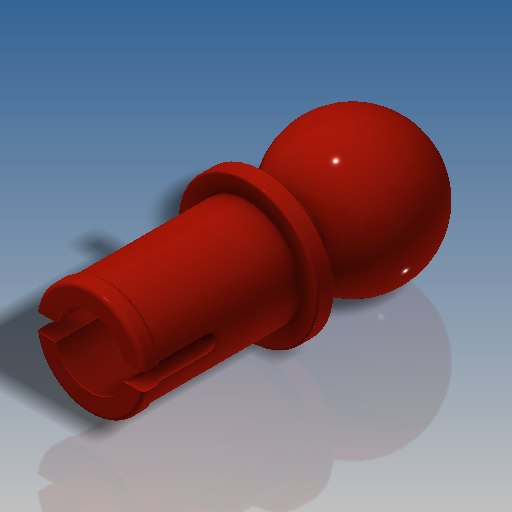
# Autodesk Inventor part: 6628-Red
Saved by Autodesk Inventor 2019.4 (Build 234330000, 330)
## iProperties
Created: 2014-06-03
Part Number: 6628-Red
Material: ABS Plastic
Document SubType Name: Modeling
Designer: D. Kohfeld
Appearance: Red
Density: 1.06 g/cm^3
Mass: 0.254458 g
Surface Area: 3.85266 cm^2
Volume: 0.240054 cm^3
Author: D. Kohfeld
Autodesk Inventor part; units mm, degrees
ref_plane "YZ Plane" through (0, 0, 0) normal (1, 0, 0) x (0, 1, 0)
ref_plane "XZ Plane" through (0, 0, 0) normal (0, 1, 0) x (-1, 0, 0)
ref_plane "XY Plane" through (0, 0, 0) normal (0, 0, 1) x (1, 0, 0)
sketch "Sketch1" plane through (0, 0, 0) normal (0, 1, 0) x (-1, 0, 0)
  line L0 (2.4, 7.2) -> (2.4, 0.8)
  line L1 (3.2, 0.8) -> (2.4, 0.8)
  line L2 (3.2, 0.8) -> (3.2, 0)
  line L3 (2.5, 8) -> (2.5, 7.2)
  line L4 (2.5, 8) -> (1.6, 8)
  line L5 (0, -10.9766) -> (0, 11.1628) projected
  line L6 (2.4, 7.2) -> (2.5, 7.2)
  line L7 (1.6, 8) -> (1.6, 0.8)
  line L8 (4.6692, 0) -> (-0.7782, 0) projected
  line L9 (1.6, 0.8) -> (0, 0.8)
  line L10 (0, -7.2) -> (0, 0.8)
  line L11 (3.2, 0) -> (1.6, 0)
  line L12 (1.6, 0) -> (1.6, -1.2287)
  arc A0 (0, -7.2) -> (1.6, -1.2287) centre (0, -4) ccw
  point P0 (0, 0)
  dimension "d1" = 4.8
  dimension "d2" = 5
  dimension "d6" = 8
  dimension "d7" = 0.8
  dimension "d8" = 6.4
  dimension "d9" = 0.8
  dimension "d32" = 6.4
  dimension "d33" = 4
  dimension "d34" = 3.2
  dimension "d37" = 3.2
  constraints: 22 end point, 5 point on line, 4 perpendicular, 2 point on circle, 1 centre point, 1 horizontal alignment, 1 parallel
  measures "d1" diameter of L0 L5
  measures "d2" diameter of L3 L5
  measures "d6" distance between parallel lines of L4 L8
  measures "d7" distance from line of L3.end L4
  measures "d8" diameter of L2 L5
  measures "d9" distance between parallel lines of L1 L8
  measures "d32" diameter of A0
  measures "d33" distance from line of L8 A0.centre
  measures "d34" diameter of L12 L5
  measures "d37" diameter of L7 L5
revolve "Revolution1" add sketch "Sketch1" angle 360 about axis through (0, 0, -10) along (0, 0, 1)
fillet "Fillet1" radius 0.2 2 edges at (2.5, 0, 8) (2.5, 0, 7.2)
fillet "Fillet1" radius 0.1 2 edges at (3.2, 0, 0) (3.2, 0, 0.8)
sketch "Sketch2" plane through (0, 0, 0) normal (1, 0, 0) x (0, 1, 0)
  line L0 (-1.6, 8) -> (1.6, 8) projected
  line L1 (-0.4, 8) -> (0.4, 8)
  line L2 (0.4, 8) -> (0.4, 5)
  line L3 (-0.4, 5) -> (-0.4, 8)
  arc A0 (-0.4, 5) -> (0.4, 5) centre (0, 5) ccw
  point P0 (0, 0)
  point P1 (0, 8)
  dimension "d35" = 3.4
  dimension "d36" = 0.8
  constraints: 6 end point, 2 midpoint, 2 point on circle, 2 tangent, 1 centre point, 1 horizontal, 1 parallel, 1 perpendicular, 1 point on line
  measures "d36" diameter of A0
extrude "Extrusion2" cut sketch "Sketch2" along normal through all both and the other way through all
equation "\"d1\" = tpd"
equation "\"d2\" = tpcd"
equation "\"d6\" = d19"
equation "\"d7\" = d9"
equation "\"d8\" = tsd"
equation "\"d9\" = tsl"
equation "\"d33\" = 0.5 * lu"
equation "\"d34\" = 0.333333 * lh"
equation "\"d37\" = rd"
equation "\"d27\" = pinf"
equation "\"d28\" = lf"
equation "\"d35\" = tpnl"
equation "\"d36\" = tpnw"
equation "\"tpd\" = 4.8"
equation "\"tpcd\" = 5"
equation "\"d19\" = 8"
equation "\"tsd\" = 6.4"
equation "\"tsl\" = 0.8"
equation "\"lu\" = 8"
equation "\"lh\" = 9.6"
equation "\"rd\" = 3.2"
equation "\"pinf\" = 0.2"
equation "\"lf\" = 0.1"
equation "\"tpnl\" = 3.4"
equation "\"tpnw\" = 0.8"
body "Solid2"
